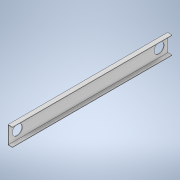
# Autodesk Inventor part: VerseFrameCChannel 18in
Saved by Autodesk Inventor 2021.1 (Build 251245000, 245)
## iProperties
Created: 2021-02-26
Part Number: VerseFrameCChannel 18in
Material: Generic
Document SubType Name: Modeling
Designer: Merkileg
Density: 1 g/cm^3
Appearance: Default
Author: Merkileg
Autodesk Inventor part; units mm, degrees
ref_plane "YZ Plane" through (0, 0, 0) normal (1, 0, 0) x (0, 1, 0)
ref_plane "XZ Plane" through (0, 0, 0) normal (0, 1, 0) x (-1, 0, 0)
ref_plane "XY Plane" through (0, 0, 0) normal (0, 0, 1) x (1, 0, 0)
sketch "Sketch1" plane through (0, 0, 0) normal (0, 0, 1) x (1, 0, 0)
  line L0 (0, 0) -> (12.7, 0)
  line L1 (12.7, 50.8) -> (0, 50.8)
  line L2 (0, 50.8) -> (0, 0)
  line L3 (12.7, 1.27) -> (1.27, 1.27)
  line L4 (1.27, 1.27) -> (1.27, 49.53)
  line L5 (1.27, 49.53) -> (12.7, 49.53)
  line L6 (12.7, 0) -> (12.7, 1.27)
  line L7 (12.7, 49.53) -> (12.7, 50.8)
  dimension "d0" = 12.7
  dimension "d1" = 50.8
  dimension "d2" = 11.43
  dimension "d3" = 48.26
  constraints: 16 end point, 6 perpendicular, 3 parallel, 1 horizontal
  measures "d0" distance of L1.end L1.start
  measures "d1" distance of L1.start L0.end
  measures "d2" distance of L3.start L3.end
  measures "d3" distance of L3.end L4.end
extrude "Extrusion1" add sketch "Sketch1" along normal blind 457.2
sketch "Sketch2" plane through (0, 0, 0) normal (-1, 0, 0) x (0, 0, 1)
  circle A0 centre (25.4, 25.4) radius 14.2875
  circle A1 centre (431.8, 25.4) radius 14.2875
  point P0 (0, 0)
  dimension "d6" = 28.575
  dimension "d7" = 28.575
  constraints: 2 centre point, 2 coincident
  measures "d6" diameter of A0
  measures "d7" diameter of A1
extrude "Extrusion2" cut sketch "Sketch2" against normal through all
equation "\"d4\" = u1"
equation "\"u1\" = 457.2"
body "Solid1"
